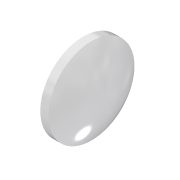
# Autodesk Inventor part: 00_Lens_f_25mm
Saved by Autodesk Inventor 2019 (Build 230136000, 136)
## iProperties
Created: 2019-08-27
Part Number: 00_Lens_f_25mm
Material: Generic
Document SubType Name: Modeling
Designer: diederichbenedict
Density: 1 g/cm^3
Appearance: Polycarbonate - Clear
Author: diederichbenedict
Autodesk Inventor part; units mm, degrees
ref_plane "YZ Plane" through (0, 0, 0) normal (1, 0, 0) x (0, 1, 0)
ref_plane "XZ Plane" through (0, 0, 0) normal (0, 1, 0) x (-1, 0, 0)
ref_plane "XY Plane" through (0, 0, 0) normal (0, 0, 1) x (1, 0, 0)
sketch "Sketch1" plane through (0, 0, 0) normal (0, 0, 1) x (1, 0, 0)
  line L0 (0, 0) -> (0, -6.34)
  line L1 (0, 0) -> (6.34, 0) construction
  line L2 (0, -6.34) -> (1.2, -6.34)
  arc A0 (1.2, -6.34) -> (3.1, 0) centre (-11.6876, 0.9769) ccw
  line L3 (0, 0) -> (3.1, 0)
  arc A1 (-1.1272, 0) -> (0, -6.34) centre (19.756, 0.4428) ccw
  line L4 (-1.1272, 0) -> (0, 0)
  line L5 (-1.1272, 0) -> (0, 0)
  dimension "d0" = 6.34
  dimension "d1" = 90
  dimension "d2" = 1.2
  dimension "d3" = 3.1
  constraints: 12 end point, 4 point on circle, 3 collinear, 2 centre point, 2 perpendicular, 1 horizontal, 1 point on line, 1 vertical
  measures "d0" distance of L0.start L0.end
  measures "d1" angle of L0 L1
  measures "d2" distance of L0.end L2.end
  measures "d3" distance of L3.end L0.start
revolve "Revolution1" add sketch "Sketch1" angle 360 about axis through (0, 0, 0) along (1, 0, 0)
body "Solid1"
